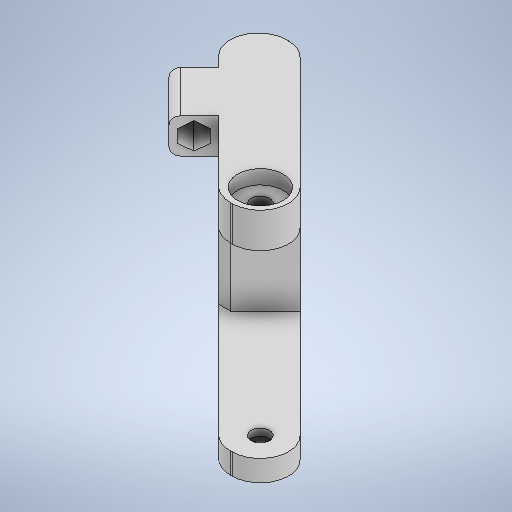
# Autodesk Inventor part: PingPongLauncherWinkel
Saved by Autodesk Inventor 2025 (Build 290162010, 162A)
## iProperties
Created: 2024-10-07
Part Number: PingPongLauncherWinkel
Material: Generisch
Document SubType Name: Modeling
Designer: max-h
Density: 1 g/cm^3
Appearance: Vorgabe
Author: max-h
Autodesk Inventor part; units mm, degrees
ref_plane "YZ Plane" through (0, 0, 0) normal (1, 0, 0) x (0, 1, 0)
ref_plane "XZ Plane" through (0, 0, 0) normal (0, 1, 0) x (-1, 0, 0)
ref_plane "XY Plane" through (0, 0, 0) normal (0, 0, 1) x (1, 0, 0)
sketch "Skizze1" plane through (0, 0, 0) normal (0, 1, 0) x (-1, 0, 0)
  line L0 (29, 0) -> (-31.1041, 60.1041)
  line L1 (0, 0) -> (29, 0)
  line L2 (-77.9249, 0) -> (46.8208, 0) projected
  line L3 (0, 0) -> (-60.1041, 60.1041)
  line L4 (-60.1041, 60.1041) -> (-31.1041, 60.1041)
  dimension "d0" = 85
  dimension "d1" = 45
  dimension "d99" = 29
  constraints: 8 end point, 2 parallel, 1 coincident, 1 point on line
  measures "d0" distance of L0.start L0.end
  measures "d1" angle of L0 L1
  measures "d99" distance of L1.start L0.start
extrude "Extrusion1" add sketch "Skizze1" along normal blind 84
fillet "Rundung2" radius 10 4 edges at (60.1041, 42, 60.1041) (31.1041, 42, 60.1041) (0, 42, 0) (-29, 42, 0)
sketch "Skizze17" plane through (0, 0, 0) normal (0, -1, 0) x (1, 0, 0)
  circle A0 centre (35.9619, 50.1041) radius 8.125
  line L0 (31.1041, 60.1041) -> (35.9619, 60.1041) projected
  line L1 (43.033, 43.033) -> (0, 0) projected
  dimension "d85" = 16.25
  dimension "d86" = 10
  dimension "d87" = 10
  constraints: 1 centre point
  measures "d85" diameter of A0
  measures "d86" distance from line of L0 A0.centre
  measures "d87" distance from line of L1 A0.centre
extrude "Extrusion18" cut sketch "Skizze17" against normal blind 5
sketch "Skizze19" plane through (0, 84, 0) normal (0, 1, 0) x (1, 0, 0)
  circle A0 centre (35.9619, -50.1041) radius 8.125 projected
  point P0 (0, 0)
  point P1 (7.3738, -32.3738)
  point P2 (4.1947, -29.1947)
  constraints: 1 other
extrude "Extrusion19" cut sketch "Skizze19" against normal blind 5
sketch "Skizze20" plane through (35.9619, 5, 50.1041) normal (0, -1, 0) x (1, 0, 0)
  circle A0 centre (0, 0) radius 3.25
  circle A1 centre (0, 0) radius 8.125 projected
  point P0 (-35.9619, -50.1041)
  point P1 (2.248, -7.6777)
  point P2 (-2.248, -7.6777)
  dimension "d96" = 6.5
  constraints: 1 centre point, 1 coincident, 1 other
  measures "d96" diameter of A0
extrude "Extrusion20" cut sketch "Skizze20" against normal through all contours A0
sketch "Skizze21" plane through (-11.9289, 0, 17.0711) normal (-0.7071068, 0, 0.7071068) x (0.7071068, 0, 0.7071068)
  line L0 (73, 71.5) -> (3, 71.5)
  line L1 (3, 71.5) -> (3, 7.5)
  line L2 (3, 7.5) -> (73, 7.5)
  line L3 (73, 7.5) -> (73, 71.5)
  line L4 (0, 84) -> (56.7157, 84) projected
  line L5 (0, 0) -> (56.7157, 0) projected
  line L6 (0, 84) -> (-7.0711, 84) projected
  line L7 (-7.0711, 84) -> (-7.0711, 0) projected
  line L8 (-7.0711, 0) -> (0, 0) projected
  line L9 (0, 0) -> (0, 84) projected
  point P0 (-3.636, 0)
  dimension "d101" = 12.5
  dimension "d102" = 7.5
  dimension "d103" = 3
  dimension "d104" = 70
  constraints: 8 end point, 2 parallel, 1 horizontal, 1 perpendicular
  measures "d101" distance between parallel lines of L4 L0
  measures "d102" distance between parallel lines of L5 L2
  measures "d103" distance between parallel lines of L1 L9
  measures "d104" distance of L1.end L2.end
extrude "Extrusion21" cut sketch "Skizze21" against normal through all contours L3 L2 L1 L0
chamfer "Fasen4" distance 3 angle 45 1 edges at (-9.8076, 39.5, 19.1924)
sketch "Skizze22" plane through (28.1751, 71.5, 57.1751) normal (-0.7071068, 0, 0.7071068) x (0.7071068, 0, 0.7071068)
  line L0 (-30.7157, 12.5) -> (-51.7157, 12.5)
  line L1 (-51.7157, 12.5) -> (-51.7157, 0)
  line L2 (-51.7157, 0) -> (-30.7157, 0)
  line L3 (-30.7157, 0) -> (-30.7157, 12.5)
  line L4 (-56.7157, 0) -> (-56.7157, 12.5) projected
  line L5 (-56.7157, 0) -> (0, 0) projected
  line L6 (-56.7157, 12.5) -> (0, 12.5) projected
  point P0 (-60.3518, -71.5)
  dimension "d110" = 21
  dimension "d118" = 5
  constraints: 8 end point, 3 collinear, 2 parallel, 1 horizontal, 1 perpendicular
  measures "d110" distance of L1.end L2.end
  measures "d118" distance between parallel lines of L4 L1
extrude "Extrusion22" add sketch "Skizze22" along normal blind 12.5 contours L3 L2 L1 L0
sketch "Skizze23" plane through (-8.3934, 71.5, 20.6066) normal (-0.7071068, 0, -0.7071068) x (-0.7071068, 0, 0.7071068)
  line L0 (2.15, 3.9117) -> (2.15, 8.5883)
  line L1 (2.15, 8.5883) -> (6.2, 10.9265)
  line L2 (6.2, 10.9265) -> (10.25, 8.5883)
  line L3 (10.25, 8.5883) -> (10.25, 3.9117)
  line L4 (10.25, 3.9117) -> (6.2, 1.5735)
  line L5 (6.2, 1.5735) -> (2.15, 3.9117)
  line L6 (12.5, 12.5) -> (12.5, 0) projected
  line L7 (12.5, 6.25) -> (3, 6.25)
  point P0 (-20.5061, -71.5)
  point P1 (6.2, 6.25)
  dimension "d114" = 8.1
  dimension "d115" = 2.25
  constraints: 14 end point, 1 horizontal, 1 midpoint, 1 parallel, 1 point on line, 13 other
  measures "d114" distance between parallel lines of L0 L3
  measures "d115" distance between parallel lines of L6 L3
extrude "Extrusion23" cut sketch "Skizze23" against normal through all
fillet "Rundung3" radius 3 2 edges at (-9.8076, 84, 36.8701) (-9.8076, 71.5, 36.8701)
